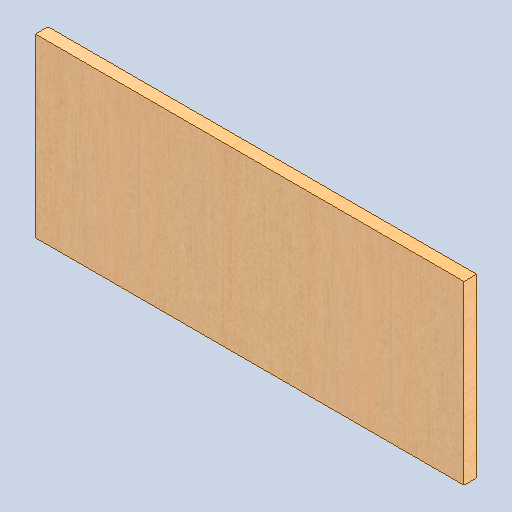
# Autodesk Inventor part: Drawer Back Panel
Saved by Autodesk Inventor 2022 (Build 260153000, 153)
## iProperties
Company: Jay's Dressers
Created: 2021-10-04
Material: Generic
Document SubType Name: Modeling
Designer: Admin
Density: 1 g/cm^3
Appearance: Yellow Pine - Solid Stained Light Low Gloss
Author: Admin
Title: Drawer Back Panel
Autodesk Inventor part; units mm, degrees
ref_plane "YZ Plane" through (0, 0, 0) normal (1, 0, 0) x (0, 1, 0)
ref_plane "XZ Plane" through (0, 0, 0) normal (0, 1, 0) x (-1, 0, 0)
ref_plane "XY Plane" through (0, 0, 0) normal (0, 0, 1) x (1, 0, 0)
sketch "Sketch1" plane through (0, 0, 0) normal (0, 0, 1) x (1, 0, 0)
  line L0 (215.9, -88.9) -> (-215.9, -88.9)
  line L1 (-215.9, -88.9) -> (-215.9, 88.9)
  line L2 (-215.9, 88.9) -> (215.9, 88.9)
  line L3 (215.9, 88.9) -> (215.9, -88.9)
  line L4 (215.9, -88.9) -> (-215.9, 88.9) construction
  line L5 (-215.9, -88.9) -> (215.9, 88.9) construction
  point P0 (0, 0)
  dimension "d0" = 431.8
  dimension "d1" = 177.8
  constraints: 12 end point, 2 midpoint, 2 parallel, 1 horizontal, 1 perpendicular
  measures "d0" distance of L1.end L2.end
  measures "d1" distance of L0.end L1.end
derived "Dresser SKELETON.ipt"
extrude "Extrusion1" add sketch "Sketch1" along normal mid plane 12.7
equation "\"d3\" = 0.5 * panelThickness"
equation "\"panelThickness\" = 25.4"
body "Solid1"
